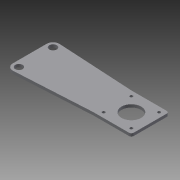
# Autodesk Inventor part: x_motor_mount
Saved by Autodesk Inventor 2013 (Build 170138000, 138)
## iProperties
Created: 2013-09-17
Part Number: x_motor_mount
Material: Generic
Document SubType Name: Modeling
Designer: Ian
Density: 1 g/cm^3
Mass: 17.922 g
Surface Area: 129.33 cm^2
Volume: 17.922 cm^3
Author: Ian
Autodesk Inventor part; units mm, degrees
ref_plane "YZ Plane" through (0, 0, 0) normal (1, 0, 0) x (0, 1, 0)
ref_plane "XZ Plane" through (0, 0, 0) normal (0, 1, 0) x (-1, 0, 0)
ref_plane "XY Plane" through (0, 0, 0) normal (0, 0, 1) x (1, 0, 0)
sketch "Sketch1" plane through (0, 0, 0) normal (0, 1, 0) x (-1, 0, 0)
  circle A0 centre (-106.68, 0) radius 11
  circle A1 centre (0, 19.05) radius 4.1656
  circle A2 centre (0, -19.05) radius 4.1656
  arc A3 (6.985, 19.05) -> (-0.3988, 26.0236) centre (0, 19.05) ccw
  arc A4 (-0.3988, -26.0236) -> (6.985, -19.05) centre (0, -19.05) ccw
  line L0 (-85.6208, 21.15) -> (-124.655, 21.15)
  line L1 (-124.655, -21.15) -> (-85.6208, -21.15)
  line L2 (-127.83, -17.975) -> (-127.83, 17.975)
  line L3 (6.985, -19.05) -> (6.985, 19.05)
  spline S0 degree 4 poles (-127.83, 17.975) (-127.83, 18.6185) (-127.83, 19.9054) (-126.5854, 21.15) (-125.2985, 21.15) (-124.655, 21.15) knots 0 0 0 0 0 0.5 1 1 1 1 1
  spline S1 degree 4 poles (-127.83, -17.975) (-127.83, -18.6185) (-127.83, -19.9054) (-126.5854, -21.15) (-125.2985, -21.15) (-124.655, -21.15) knots 0 0 0 0 0 0.5 1 1 1 1 1
  line L4 (-85.6208, 21.15) -> (-85.6208, -21.15) construction
  line L5 (-0.3988, 26.0236) -> (-85.6208, 21.15)
  line L6 (-85.6208, -21.15) -> (-0.3988, -26.0236)
  point P0 (0, 0)
  point P1 (-122.18, 15.5)
  point P2 (-91.18, 15.5)
  point P3 (-91.18, -15.5)
  point P4 (-122.18, -15.5)
  dimension "d0" = 106.68
  dimension "d1" = 19.05
  dimension "d2" = 19.05
  dimension "d5" = 22
  dimension "d8" = 8.3312
  dimension "d9" = 8.3312
  dimension "d10" = 13.97
  dimension "d11" = 13.97
  dimension "d52" = 134.815
  dimension "d53" = 42.3
  dimension "d54" = 6.985
  dimension "d55" = 21.15
  dimension "d57" = 98.165
  dimension "d59" = 98.165
  dimension "d61" = 113.665
  dimension "d62" = 129.165
  dimension "d64" = 129.165
  dimension "d66" = 131.64
  dimension "d67" = 131.64
  dimension "d70" = 3.175
  dimension "d71" = 3.175
  dimension "d72" = 5.65
  dimension "d73" = 5.65
  dimension "d74" = 5.65
  dimension "d75" = 5.65
  dimension "d76" = 93.273
  dimension "d77" = 42.3
  constraints: 14 end point, 5 centre point, 5 coincident, 4 point on circle, 4 tangent, 3 parallel, 3 vertical, 2 horizontal, 1 perpendicular, 4 other
  measures "d0" distance of point (0, 0) point (-106.68, 0)
  measures "d1" distance of point (0, 0) point (0, 19.05)
  measures "d2" distance of point (0, -19.05) point (0, 0)
  measures "d5" diameter of A0
  measures "d8" diameter of A1
  measures "d9" diameter of A2
  measures "d10" diameter of A3
  measures "d11" diameter of A4
  measures "d52" distance between parallel lines of L3 L2
  measures "d53" distance between parallel lines of L1 L0
  measures "d54" distance from line of point (0, 0) L3
  measures "d55" distance from line of point (0, 0) L0
  measures "d57" distance from line of point (-91.18, 15.5) L3
  measures "d59" distance from line of point (-91.18, -15.5) L3
  measures "d61" distance from line of point (-106.68, 0) L3
  measures "d62" distance from line of point (-122.18, 15.5) L3
  measures "d64" distance from line of point (-122.18, -15.5) L3
  measures "d66" distance from line of L0.end L3
  measures "d67" distance from line of L1.start L3
  measures "d70" horizontal distance of L0.end L2.end
  measures "d71" horizontal distance of L1.start L2.start
  measures "d72" distance from line of point (-122.18, -15.5) L1
  measures "d73" distance from line of point (-91.18, -15.5) L1
  measures "d74" distance from line of point (-122.18, 15.5) L0
  measures "d75" distance from line of point (-91.18, 15.5) L0
  measures "d76" angle of L4 L6
  measures "d77" distance of L0.start L1.end
extrude "Extrusion1" add sketch "Sketch1" along normal blind 3.175
hole "Hole1" at (106.68, 0, 0) at (0, 0, 19.05) at (0, 0, -19.05) at (122.18, 0, 15.5) at (91.18, 0, 15.5) at (91.18, 0, -15.5) at (122.18, 0, -15.5) direction (0, 1, 0) diameter 3.2004 end through all clearance for "Flat Head Machine Screw" size "M3" standard "Ansi Metric M Profile"
equation "\"d2\" = d1"
equation "\"d9\" = d8"
body "Solid1"
